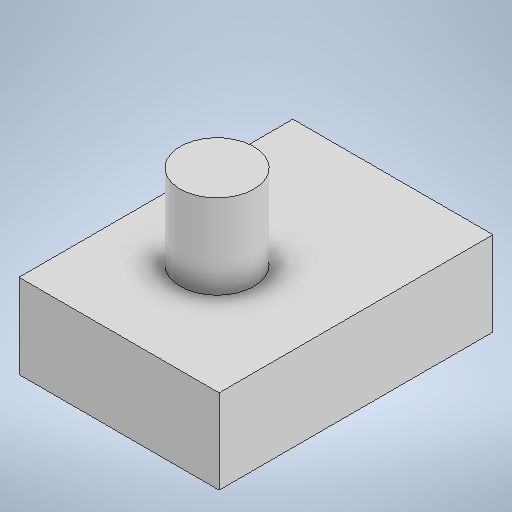
# Autodesk Inventor part: encoder
Saved by Autodesk Inventor 2025.1 (Build 291241000, 241)
## iProperties
Created: 2025-02-01
Part Number: encoder
Material: Generisch
Document SubType Name: Modeling
Designer: joebe
Density: 1 g/cm^3
Appearance: Vorgabe
Author: joebe
Autodesk Inventor part; units mm, degrees
ref_plane "YZ Plane" through (0, 0, 0) normal (1, 0, 0) x (0, 1, 0)
ref_plane "XZ Plane" through (0, 0, 0) normal (0, 1, 0) x (-1, 0, 0)
ref_plane "XY Plane" through (0, 0, 0) normal (0, 0, 1) x (1, 0, 0)
sketch "Skizze1" plane through (0, 0, 0) normal (0, 0, 1) x (1, 0, 0)
  line L0 (-9.5, 13) -> (9.5, 13)
  line L1 (9.5, 13) -> (9.5, -13)
  line L2 (9.5, -13) -> (-9.5, -13)
  line L3 (-9.5, -13) -> (-9.5, 13)
  line L4 (-9.5, 13) -> (9.5, -13) construction
  line L5 (9.5, 13) -> (-9.5, -13) construction
  point P0 (0, 0)
  dimension "d0" = 19
  dimension "d1" = 26
  constraints: 12 end point, 2 midpoint, 2 parallel, 1 horizontal, 1 perpendicular
  measures "d0" distance of L1.end L2.end
  measures "d1" distance of L0.end L1.end
extrude "Extrusion1" add sketch "Skizze1" along normal blind 8
sketch "Skizze2" plane through (0, 0, 8) normal (0, 0, 1) x (1, 0, 0)
  circle A0 centre (-1.1, -2.6) radius 3.5
  line L0 (-9.5, -13) -> (9.5, -13) projected
  line L1 (-9.5, 13) -> (-9.5, -13) projected
  point P0 (0, 0)
  dimension "d4" = 7
  dimension "d5" = 10.4
  dimension "d6" = 8.4
  constraints: 1 centre point
  measures "d4" diameter of A0
  measures "d5" distance from line of L0 A0.centre
  measures "d6" distance from line of L1 A0.centre
extrude "Extrusion2" add sketch "Skizze2" along normal blind 8
